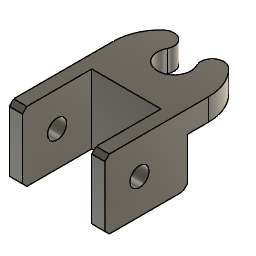
tube holder_side v1 (Autodesk Fusion 360 design; units mm, degrees)
Autodesk Fusion 360 part; units mm, degrees
note: some values were not read from the file. Set by a fixed rule: which sketch regions a step uses.
sketch "Sketch1" plane through (0, 0, 0) normal (0, 0, 1) x (1, 0, 0)
  line L0 (0, 0) -> (3.81, 0)
  line L1 (3.81, 0) -> (3.81, 20)
  line L2 (3.81, 20) -> (23.81, 20)
  line L3 (23.81, 20) -> (23.81, 0)
  line L4 (23.81, 0) -> (27.62, 0)
  line L5 (27.62, 0) -> (27.62, 23.81)
  line L6 (27.62, 23.81) -> (0, 23.81)
  line L7 (0, 23.81) -> (0, 0)
  dimension "d1" = 3.81
  dimension "d2" = 20
  dimension "d3" = 3.81
  constraint coincident L0.start L7.end
  constraint horizontal L0
  constraint perpendicular L0 L1
  constraint perpendicular L1 L2
  constraint perpendicular L2 L3
  constraint perpendicular L1 L4
  constraint perpendicular L2 L5
  constraint perpendicular L5 L6
  constraint vertical L7
  constraint equal L0 L4
  constraint equal L1 L2
  measures "d1" distance of L0.start L0.end
  measures "d2" distance of L1.end L2.end
  measures "d3" distance of L2 L6
extrude "Extrude1" add sketch "Sketch1" against normal blind 20
sketch "Sketch2" plane through (0, 0, 0) normal (0, 0, 1) x (-1, 0, 0)
  line L0 (0, -23.81) -> (0, 0)
  circle A0 centre (-13.81, -33.81) radius 4.8
  line L1 (-27.62, -23.81) -> (0, -23.81)
  line L2 (-13.81, -43.81) -> (-13.81, -33.81) construction
  line L3 (-13.81, -33.81) -> (-13.81, -23.81) construction
  line L4 (-27.62, -23.81) -> (-27.62, -30)
  line L5 (0, -23.81) -> (0, -30)
  arc A1 (-27.62, -30) -> (0, -30) centre (-13.81, -30) ccw
  line L6 (-3.81, -20) -> (-23.81, -20)
  point P0 (-27.62, -23.81)
  point P1 (0, -23.81)
  dimension "d6" = 9.6
  dimension "d25" = 10
  constraint coincident P0 L1.start
  constraint coincident P1 L0.start
  constraint coincident A0.centre L2.end
  constraint equal L2 L3
  constraint perpendicular L1 L4
  constraint perpendicular L1 L5
  constraint horizontal L4.end L5.end
  constraint tangent L5 A1
  constraint coincident L2.start A1
  constraint coincident L1 L3.end
  constraint vertical A0.centre L2.start
  constraint vertical A0.centre L3.end
  constraint midpoint L2.start A1
  measures "d6" diameter of A0
  measures "d25" distance of A0.centre L1
extrude "Extrude2" add sketch "Sketch2" against normal blind 6.35
sketch "Sketch3" plane through (27.62, 0, 0) normal (1, 0, 0) x (0, 1, 0)
  line L0 (0, 0) -> (0, -20)
  line L1 (0, -10) -> (10, -10)
  dimension "d10" = 10
  constraint midpoint L0 L1.start
  constraint perpendicular L0 L1
  measures "d10" distance of L1.start L1.end
hole "Hole1" at (27.62, 10, -10) direction (-1, 0, 0) diameter 5.5118 depth 116.84 tip angle 118
chamfer "Chamfer1" distance 1.27 angle 45 4 edges at (25.715, 0, 0) (25.715, 0, -20) (1.905, 0, -20) (1.905, 0, 0)
chamfer "Chamfer2" distance 1.27 angle 45 1 edges at (13.81, 23.81, -20)
sketch "Sketch4" plane through (0, 0, 0) normal (0, 0, 1) x (-1, 0, 0)
  arc A0 (-27.62, -30) -> (0, -30) centre (-13.81, -30) ccw
  circle A1 centre (-13.81, -33.81) radius 4.8
  arc A2 (-9.569, -36.0581) -> (-4.334, -40.046) centre (-6.6224, -37.62) ccw
  arc A3 (-23.286, -40.046) -> (-18.051, -36.0581) centre (-20.9976, -37.62) ccw
  dimension "d20" = 3.81
  constraint tangent A1 A2
  constraint coincident A0 A2.end
  constraint coincident A1 A2.start
  constraint tangent A0 A2
  constraint tangent A1 A3
  constraint coincident A0 A3.start
  constraint tangent A0 A3
  constraint horizontal A2.start A3.end
  constraint horizontal A2.end A3.start
  measures "d20" vertical distance of A1.centre A2.centre
extrude "Extrude3" cut sketch "Sketch4" against normal blind 11.43 contours A0 A1 A2 A3
